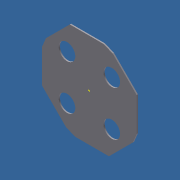
# Autodesk Inventor part: Stage2
Saved by Autodesk Inventor 2018 (Build 220112000, 112)
## iProperties
Created: 2018-10-31
Part Number: Stage2
Material: 3.3547 AlMg4,5Mn (AW-5083/H111)
Document SubType Name: Modeling
Designer: N.Grubert
Density: 2.66 g/cm^3
Appearance: Aluminum (gleichmäßig)
Fläche: 0 cm²
Gewicht: 0 g
Material: geeigneten Werkstoff auswählen !
Dateiname: P:\INVENTOR\Inventor 2018\Templates\ILT\Norm.ipt
Bez_eng: bolt
Bez_french: boulon
Author: N.Grubert
Autodesk Inventor part; units mm, degrees
ref_plane "YZ Plane" through (0, 0, 0) normal (1, 0, 0) x (0, 1, 0)
ref_plane "XZ Plane" through (0, 0, 0) normal (0, 1, 0) x (-1, 0, 0)
ref_plane "XY Plane" through (0, 0, 0) normal (0, 0, 1) x (1, 0, 0)
sketch "Skizze4" plane through (0, 0, 0) normal (0, 1, 0) x (-1, 0, 0)
  line L0 (-23.6102, 57) -> (23.6102, 57)
  line L1 (23.6102, 57) -> (57, 23.6102)
  line L2 (57, 23.6102) -> (57, -23.6102)
  line L3 (57, -23.6102) -> (23.6102, -57)
  line L4 (23.6102, -57) -> (-23.6102, -57)
  line L5 (-23.6102, -57) -> (-57, -23.6102)
  line L6 (-57, -23.6102) -> (-57, 23.6102)
  line L7 (-57, 23.6102) -> (-23.6102, 57)
  line L8 (79.8, 0) -> (-79.8, 0) construction
  line L9 (0, -79.8) -> (0, 79.8) construction
  circle A0 centre (-27, 27) radius 10
  circle A1 centre (-27, -27) radius 10
  circle A2 centre (27, -27) radius 10
  circle A3 centre (27, 27) radius 10
  point P0 (0, 0)
  point P1 (0, 0)
  dimension "d4" = 114
  dimension "d5" = 20
  dimension "d6" = 30
  dimension "d7" = 30
  dimension "d10" = 360
  constraints: 16 end point, 4 centre point, 1 coincident, 28 other
  measures "d4" distance between parallel lines of L4 L0
  measures "d5" diameter of A0
  measures "d6" distance from line of A0.centre L6
  measures "d7" distance from line of A0.centre L0
extrude "Extrusion2" add sketch "Skizze4" along normal blind 2.5
sketch "Skizze5" plane through (0, 0, 0) normal (0, -1, 0) x (1, 0, 0)
  circle A0 centre (-27, 27) radius 10 construction
  circle A1 centre (-27, -27) radius 10 construction
  circle A2 centre (27, -27) radius 10 construction
  circle A3 centre (27, 27) radius 10 construction
  line L0 (23.6102, 57) -> (-23.6102, 57) construction
  line L1 (-23.6102, 57) -> (-57, 23.6102) construction
  line L2 (-57, 23.6102) -> (-57, -23.6102) construction
  line L3 (-57, -23.6102) -> (-23.6102, -57) construction
  line L4 (-23.6102, -57) -> (23.6102, -57) construction
  line L5 (23.6102, -57) -> (57, -23.6102) construction
  line L6 (57, -23.6102) -> (57, 23.6102) construction
  line L7 (57, 23.6102) -> (23.6102, 57) construction
  line L8 (23.6102, 57) -> (57, 23.6102) construction
  line L9 (-57, -23.6102) -> (-57, 23.6102) construction
  line L10 (-23.6102, -57) -> (-57, -23.6102) construction
  line L11 (23.6102, -57) -> (-23.6102, -57) construction
  line L12 (57, 23.6102) -> (57, -23.6102) construction
  line L13 (-57, 17.1158) -> (-52.4078, 28.2024)
  line L14 (-57, 23.6102) -> (-23.6102, 57) projected
  line L15 (-57, 23.6102) -> (-57, -23.6102) projected
  line L16 (-57, 23.6102) -> (-52.4078, 28.2024)
  line L17 (-23.6102, 57) -> (-57, 23.6102) projected
  line L18 (-57, 23.6102) -> (-57, 17.1158)
  line L19 (-23.6102, -57) -> (-28.2024, -52.4078)
  line L20 (-17.1158, -57) -> (-28.2024, -52.4078)
  line L21 (-23.6102, -57) -> (-17.1158, -57)
  line L22 (57, -23.6102) -> (52.4078, -28.2024)
  line L23 (57, -17.1158) -> (52.4078, -28.2024)
  line L24 (57, -23.6102) -> (57, -17.1158)
  line L25 (23.6102, 57) -> (28.2024, 52.4078)
  line L26 (17.1158, 57) -> (28.2024, 52.4078)
  line L27 (23.6102, 57) -> (17.1158, 57)
  point P0 (0, 0)
  dimension "d21" = 22.5
  dimension "d22" = 12
  dimension "d25" = 360
  constraints: 24 end point, 4 coincident, 2 collinear, 2 point on line, 25 other
  measures "d21" angle of L13 L1
  measures "d22" distance of L13.start L13.end
extrude "Extrusion3" cut sketch "Skizze5" against normal blind 10
sketch "Skizze6" plane through (0, 2.5, 0) normal (0, 1, 0) x (1, 0, 0)
  line L0 (57, 17.1158) -> (52.4078, 28.2024) projected
  line L1 (52.4078, 28.2024) -> (23.6102, 57) projected
  line L2 (23.6102, 57) -> (-17.1158, 57) projected
  line L3 (-17.1158, 57) -> (-28.2024, 52.4078) projected
  line L4 (-28.2024, 52.4078) -> (-57, 23.6102) projected
  line L5 (-57, 23.6102) -> (-57, -17.1158) projected
  line L6 (-57, -17.1158) -> (-52.4078, -28.2024) projected
  line L7 (-52.4078, -28.2024) -> (-23.6102, -57) projected
  line L8 (-23.6102, -57) -> (17.1158, -57) projected
  line L9 (17.1158, -57) -> (28.2024, -52.4078) projected
  line L10 (28.2024, -52.4078) -> (57, -23.6102) projected
  line L11 (57, -23.6102) -> (57, 17.1158) projected
  circle A0 centre (-27, -27) radius 10 projected
  circle A1 centre (-27, 27) radius 10 projected
  circle A2 centre (27, 27) radius 10 projected
  circle A3 centre (27, -27) radius 10 projected
  point P0 (0, 0)
extrude "Extrusion4" cut sketch "Skizze6" against normal blind 1
sketch "Skizze7" plane through (0, 0, 0) normal (0, -1, 0) x (1, 0, 0)
  line L0 (52.4078, -28.2024) -> (57, -17.1158) construction
  line L1 (57, -17.1158) -> (57, 23.6102) construction
  line L2 (57, 23.6102) -> (28.2024, 52.4078) construction
  line L3 (28.2024, 52.4078) -> (17.1158, 57) construction
  line L4 (17.1158, 57) -> (-23.6102, 57) construction
  line L5 (-23.6102, 57) -> (-52.4078, 28.2024) construction
  line L6 (-52.4078, 28.2024) -> (-57, 17.1158) construction
  line L7 (-57, 17.1158) -> (-57, -23.6102) construction
  line L8 (-57, -23.6102) -> (-28.2024, -52.4078) construction
  line L9 (-28.2024, -52.4078) -> (-17.1158, -57) construction
  line L10 (-17.1158, -57) -> (23.6102, -57) construction
  line L11 (23.6102, -57) -> (52.4078, -28.2024) construction
  circle A0 centre (-27, 27) radius 10 construction
  circle A1 centre (-27, -27) radius 10 construction
  circle A2 centre (27, -27) radius 10 construction
  circle A3 centre (27, 27) radius 10 construction
  line L12 (-37, 27) -> (-37, -27)
  circle A4 centre (-27, -27) radius 10 projected
  line L13 (-17, -27) -> (-17, 27)
  line L14 (37, -27) -> (37, 27)
  line L15 (17, -27) -> (17, 27)
  circle A5 centre (27, 27) radius 10 projected
  arc A6 (-17, 27) -> (-37, 27) centre (-27, 27) ccw
  arc A7 (37, 27) -> (17, 27) centre (27, 27) ccw
  circle A8 centre (27, -27) radius 10 projected
  arc A9 (17, -27) -> (37, -27) centre (27, -27) ccw
  circle A10 centre (-27, -27) radius 10 projected
  arc A11 (-37, -27) -> (-17, -27) centre (-27, -27) ccw
  point P0 (0, 0)
  constraints: 19 point on circle, 8 end point, 8 tangent, 4 centre point, 2 parallel, 2 vertical, 1 point on line
extrude "Extrusion5" cut sketch "Skizze7" against normal through all
equation "\"d7\" = d6"
